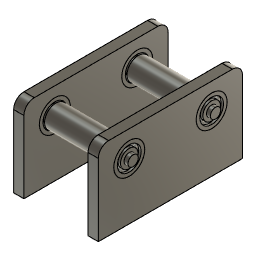
2gear-box (Autodesk Fusion 360 design; units mm, degrees)
Autodesk Fusion 360 part; units mm, degrees
sketch "Wall1" plane through (0, 0, 0) normal (1, 0, 0) x (0, 1, 0) in component "Wall1"
  line L0 (400, 300) -> (-800, 300)
  line L1 (-900, 200) -> (-900, -500)
  line L2 (-900, -500) -> (500, -500)
  line L3 (500, -500) -> (500, 200)
  arc A0 (500, 200) -> (400, 300) centre (400, 200) ccw
  arc A1 (-800, 300) -> (-900, 200) centre (-800, 200) ccw
  circle A2 centre (200, 50) radius 150
  circle A3 centre (-600, 50) radius 150
  dimension "d1" = 100
  dimension "d2" = 100
  constraint horizontal L0
  constraint vertical L1
  constraint horizontal L2
  constraint vertical L3
  constraint tangent L0 A0
  constraint tangent L3 A0
  constraint tangent L1 A1
  constraint tangent L0 A1
  measures "d1" radius of A0
  measures "d2" radius of A1
extrude "Extrude1" add sketch "Wall1" against normal blind 200 makes body 1 in component "Wall1"
move_body "Move1" bodies 1 to x (1, 0, 0) y (0, 1, 0) z (0, 0, 1) at (-500, 0, 0) in component "Wall1"
move_body "Move2" bodies 1 to x (1, 0, 0) y (0, 1, 0) z (0, 0, 1) at (-200, 0, 0) in component "Wall1"
move_body "Move3" bodies 1 to x (1, 0, 0) y (0, 1, 0) z (0, 0, 1) at (0, 200, 0) in component "Wall1"
sketch "Wall2" plane through (0, 0, 0) normal (1, 0, 0) x (0, 1, 0) in component "Wall2"
  line L0 (-700, -500) -> (700, -500)
  line L1 (700, -500) -> (700, 200)
  line L2 (600, 300) -> (-600, 300)
  line L3 (-700, 200) -> (-700, -500)
  arc A0 (700, 200) -> (600, 300) centre (600, 200) ccw
  arc A1 (-600, 300) -> (-700, 200) centre (-600, 200) ccw
  circle A2 centre (-400, 50) radius 150
  circle A3 centre (400, 50) radius 150
  dimension "d7" = 100
  dimension "d8" = 100
  constraint horizontal L0
  constraint vertical L1
  constraint horizontal L2
  constraint vertical L3
  constraint tangent L1 A0
  constraint tangent L2 A0
  constraint tangent L2 A1
  constraint tangent L3 A1
  measures "d7" radius of A0
  measures "d8" radius of A1
extrude "Extrude1'" add sketch "Wall2" along normal blind 200 separate body makes body 2 in component "Wall2"
move_body "Move1'" bodies 2 to x (1, 0, 0) y (0, 1, 0) z (0, 0, 1) at (700, 0, 0) in component "Wall2"
sketch "Rulment" plane through (0, 0, 0) normal (0, 1, 0) x (1, 0, 0) in component "Bearing"
  line L0 (0, 0) -> (150, 0)
  line L1 (150, 0) -> (-150, 0)
  line L2 (50, -150) -> (-50, -150)
  line L3 (-50, -150) -> (-50, -115)
  line L4 (50, -115) -> (50, -150)
  line L5 (-50, -50) -> (-50, -85)
  line L6 (50, -85) -> (50, -50)
  line L7 (50, -50) -> (-50, -50)
  circle A0 centre (0, -100) radius 30
  line L8 (-50, -115) -> (-25.9808, -115)
  line L9 (25.9808, -115) -> (50, -115)
  line L10 (-50, -85) -> (-25.9808, -85)
  line L11 (25.9808, -85) -> (50, -85)
  line L12 (0, -150) -> (0, -50)
  constraint coincident L0.start origin
  constraint horizontal L2
  constraint vertical L3
  constraint horizontal L8
  constraint vertical L4
  constraint coincident A0 L8.end
  constraint coincident A0 L9.start
  constraint collinear L8 L9
  constraint coincident A0 L10.end
  constraint coincident A0 L11.start
  constraint collinear L10 L11
  constraint midpoint L2 L12.start
  constraint midpoint L7 L12.end
  constraint perpendicular L7 L12
revolve "Revolve1" add sketch "Rulment" angle 360 about axis through (150, 0, 0) along (-1, 0, 0) separate body contours L2 L4 A0 L9 L12 | L2 L3 A0 L8 L12 | L6 L7 A0 L11 L12 | L5 L7 A0 L10 L12 makes body 3 at (16.6667, -7.4769, 149.8135) makes body 4 at (16.6667, -2.4923, 49.9378) in component "Bearing"
revolve "Revolve2" add sketch "Rulment" angle 360 about axis through (0, 0, 150) along (0, 0, -1) separate body contours A0 L12 picked at (18.9881, -106.052) makes body 5 in component "Bearing"
pattern_circular "C-Pattern1" count 10 over 360 about axis through (1.75, 0, 0) along (1, 0, 0) of bodies 5 makes body 6 at (-6.3404, -37.2713, 100.8326) makes body 7 at (-6.3404, -89.421, 59.6677) makes body 8 at (-28.3843, -101.2196, -23.3553) makes body 9 at (-6.3404, -84.38, -66.6061) makes body 10 at (28.3843, -9.0664, -103.4828) makes body 11 at (22.0439, 44.6062, -95.5035) makes body 12 at (-6.3404, 89.421, -59.6677) makes body 13 at (28.3843, 95.6163, 40.6006) makes body 14 at (-6.3404, 84.38, 66.6061) in component "Bearing"
extrude "Extrude2" cut 1 faces at (-900, 108.3333, -359.9679) along direction (1, 0, 0) blind 100 on bodies 1 bodies 1 in component "Wall1"
extrude "Extrude2'" cut 1 faces at (900, 108.3333, -359.9679) along direction (-1, 0, 0) blind 100 on bodies 2 bodies 2 in component "Wall2"
sketch "ax" plane through (0, 0, 0) normal (1, 0, 0) x (0, 1, 0) in component "Ax1"
  circle A0 centre (400, 0) radius 50
  circle A1 centre (400, 0) radius 110
extrude "Extrude2''" add sketch "ax" along normal mid plane 900 separate body contours A0 makes body 15 in component "Ax1"
extrude "Extrude3" add sketch "ax" along normal mid plane 600 bodies 15 in component "Ax1"
sketch "ax (2)" plane through (0, 0, 0) normal (1, 0, 0) x (0, 1, 0) in component "Ax2"
  circle A0 centre (-400, 0) radius 50
  circle A1 centre (-400, 0) radius 110
extrude "Extrude1''" add sketch "ax (2)" along normal mid plane 900 separate body contours A0 makes body 16 in component "Ax2"
extrude "Extrude2'''" add sketch "ax (2)" along normal mid plane 600 bodies 16 in component "Ax2"
component "Big_Gear1" placed x (1, 0, 0) y (0, 1, 0) z (0, 0, 1) at (0, 0, 0)
component "Big_Gear2" placed x (1, 0, 0) y (0, 1, 0) z (0, 0, 1) at (0, 0, 0)
component "Small_Gear1" placed x (1, 0, 0) y (0, 1, 0) z (0, 0, 1) at (0, 0, 0)
component "Small_gear2" placed x (1, 0, 0) y (0, 1, 0) z (0, 0, 1) at (0, 0, 0)
component "Wall1" placed x (1, 0, 0) y (0, 1, 0) z (0, 0, 1) at (0, 0, -50)
component "Wall2" placed x (1, 0, 0) y (0, 1, 0) z (0, 0, 1) at (0, 0, -50)
component "Ax1" placed x (1, 0, 0) y (0, 1, 0) z (0, 0, 1) at (0, 0, 0)
component "Ax2" placed x (1, 0, 0) y (0, 1, 0) z (0, 0, 1) at (0, 0, 0)
component "Ring" placed x (1, 0, 0) y (0, 1, 0) z (0, 0, 1) at (0, 0, 0)
component "Link1" placed x (1, 0, 0) y (0, 1, 0) z (0, 0, 1) at (0, 0, 0)
component "Link2" placed x (1, 0, 0) y (0, 1, 0) z (0, 0, 1) at (0, 0, 0)
component "Lever" placed x (1, 0, 0) y (0, 1, 0) z (0, 0, 1) at (0, 0, 0)
component "Bearing" placed x (-1, 0, 0) y (0, 0, 1) z (0, 1, 0) at (-750, -400, 0)
component "Bearing" placed x (1, 0, 0) y (0, 1, 0) z (0, 0, 1) at (-750, 400, 0)
component "Bearing" placed x (1, 0, 0) y (0, 0, -1) z (0, 1, 0) at (750, 400, 0)
component "Bearing" placed x (-1, 0, 0) y (0, 1, 0) z (0, 0, -1) at (750, -400, 0)
named bodies: "Wall1", "Wall2", "Outer-circle", "Inner-circle", "bila 10", "bila 1", "bila 2", "bila 3", "bila 4", "bila 5", "bila 6", "bila 7", "bila 8", "bila 9", "ax"
